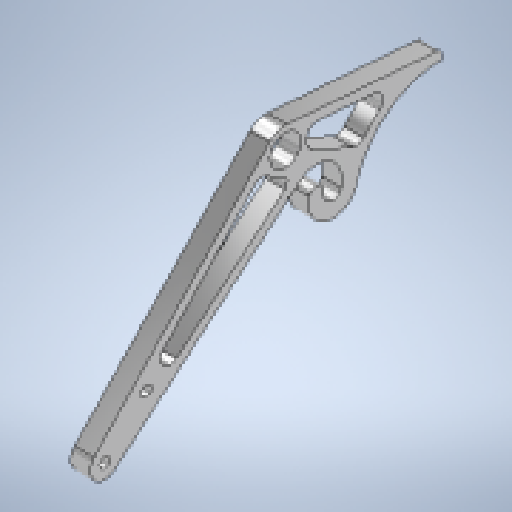
# Autodesk Inventor part: Arm
Saved by Autodesk Inventor 2023.2 (Build 272271000, 271)
## iProperties
Created: 2023-08-22
Part Number: Arm
Material: Aluminum 6061
Document SubType Name: Modeling
Designer: Nathan Cai
Mass: 24.1301 g
Surface Area: 65.2263 cm^2
Volume: 8.93708 cm^3
Density: 2.7 g/cm^3
Appearance: Aluminum - Flat
Author: Nathan Cai
Autodesk Inventor part; units mm, degrees
ref_plane "YZ Plane" through (0, 0, 0) normal (1, 0, 0) x (0, 1, 0)
ref_plane "XZ Plane" through (0, 0, 0) normal (0, 1, 0) x (-1, 0, 0)
ref_plane "XY Plane" through (0, 0, 0) normal (0, 0, 1) x (1, 0, 0)
sketch "Sketch1" plane through (0, 0, 0) normal (1, 0, 0) x (0, 1, 0)
  circle A0 centre (28.575, 50.8) radius 7
  circle A1 centre (0, 0) radius 28.575
  line L0 (0, 0) -> (28.575, 50.8) construction
  line L1 (28.575, 0) -> (-28.575, 0)
  arc A2 (13.9234, 2.1588) -> (28.575, 0) centre (28.575, 50.8) ccw construction
  line L2 (28.575, 0) -> (28.575, 43.8) construction
  circle A3 centre (28.575, 50.8) radius 5
  circle A4 centre (30.1625, 1.5875) radius 1.5875
  line L3 (30.1625, 0) -> (28.575, 0)
  line L4 (31.7452, 1.464) -> (35.5538, 50.2552)
  circle A5 centre (-28.575, 87.3125) radius 3 construction
  line L5 (23.4933, 45.9858) -> (-33.7928, 106.4549) construction
  line L6 (33.3896, 55.8813) -> (-26.8868, 112.9946)
  arc A6 (10.9573, 40.6232) -> (8.0927, 30.0027) centre (9.525, 35.313) ccw construction
  arc A7 (11.6084, 43.0369) -> (7.4416, 27.589) centre (9.525, 35.313) ccw
  arc A8 (10.3063, 38.2094) -> (8.7437, 32.4165) centre (9.525, 35.313) ccw
  arc A9 (10.3063, 38.2094) -> (11.6084, 43.0369) centre (10.9573, 40.6232) ccw
  arc A10 (7.4416, 27.589) -> (8.7437, 32.4165) centre (8.0927, 30.0027) ccw construction
  arc A11 (9.525, 35.313) -> (15.1497, 44.1832) centre (10.9573, 40.6232) ccw construction
  arc A12 (8.7437, 32.4165) -> (17.4365, 46.125) centre (10.9573, 40.6232) ccw
  arc A13 (10.3063, 38.2094) -> (12.863, 42.2414) centre (10.9573, 40.6232) ccw
  arc A14 (10.3063, 38.2094) -> (8.7437, 32.4165) centre (9.525, 35.313) ccw
  arc A15 (17.4365, 46.125) -> (12.863, 42.2414) centre (15.1497, 44.1832) ccw construction
  line L7 (17.4365, 46.125) -> (-33.7928, 106.4549)
  line L8 (9.525, 35.313) -> (-28.575, 87.3125) construction
  arc A16 (-26.8868, 112.9946) -> (-33.7928, 106.4549) centre (-30.1625, 109.5375) ccw
  line L9 (-25.4, 109.5375) -> (-34.925, 109.5375) construction
  circle A17 centre (-30.1625, 109.5375) radius 1.7526
  line L10 (28.575, 50.8) -> (-30.1625, 109.5375) construction
  circle A18 centre (-16.6921, 96.0671) radius 1.7526
  circle A19 centre (-16.6921, 96.0671) radius 5.2756
  line L11 (26.9502, 57.6088) -> (-11.7344, 94.2634)
  line L12 (-16.3371, 90.8034) -> (17.5275, 50.9231)
  arc A20 (17.5275, 50.9231) -> (21.6861, 52.0419) centre (19.3426, 52.4644) ccw
  line L13 (29.3849, 12.0246) -> (31.9322, 44.6576)
  arc A21 (29.3849, 12.0246) -> (2.4085, 31.6585) centre (0, 0) ccw
  arc A22 (31.7234, 1.2983) -> (31.6845, 2.0389) centre (0, 0) ccw
  line L14 (17.3128, 26.6145) -> (25.6201, 44.4543)
  circle A23 centre (20.102, 36.3649) radius 1.5875 construction
  line L15 (10.9573, 40.6232) -> (20.102, 36.3649) construction
  point P0 (-20.3953, 106.8437)
  point P1 (8.7437, 32.4165)
  point P2 (7.4416, 27.589)
  point P3 (12.863, 42.2414)
  dimension "d0" = 14
  dimension "d1" = 57.15
  dimension "d3" = 50.8
  dimension "d4" = 10
  dimension "d5" = 3.175
  dimension "d6" = 6
  dimension "d13" = 2.5
  dimension "d15" = 19.05
  dimension "d21" = 3
  dimension "d25" = 57.15
  dimension "d30" = 9.525
  dimension "d33" = 63.5
  dimension "d34" = 22.225
  dimension "d35" = 64.4637
  dimension "d36" = 3.5052
  dimension "d37" = 45
  dimension "d40" = 19.05
  dimension "d45" = 3.175
  dimension "d46" = 3.175
  dimension "d47" = 4.7625
  dimension "d48" = 3.175
  dimension "d50" = 3.175
  dimension "d51" = 3.175
  constraints: 43 point on circle, 32 end point, 24 tangent, 23 centre point, 6 coincident, 4 point on line, 3 midpoint, 3 perpendicular, 1 horizontal, 1 parallel, 17 other
  measures "d1" diameter of A1
  measures "d3" vertical distance of point (0, 0) L0.end
  measures "d4" diameter of A3
  measures "d5" diameter of A4
  measures "d6" diameter of A5
  measures "d13" radius of A9
  measures "d15" horizontal distance of L10.start L8.start
  measures "d21" radius of A8
  measures "d25" horizontal distance of L10.start L8.end
  measures "d30" diameter of A16
  measures "d33" horizontal distance of L10.start L9.end
  measures "d34" distance from line of L9 L8.end
  measures "d35" distance of L8.start L8.end
  measures "d36" diameter of A17
  measures "d37" angle of L2 L10
  measures "d40" distance of L10.end A18.centre
  measures "d45" distance between parallel lines of L6 L11
  measures "d46" distance between parallel lines of L7 L12
  measures "d47" diameter of A20
  measures "d48" distance between parallel lines of L4 L13
  measures "d50" radial gap between concentric circles of A1 A21
  measures "d51" diameter of A23
extrude "Extrusion1" add sketch "Sketch1" along normal blind 6.35 contours A0 | A0 L11 A19 L6 | L4 A4 L3 A1 A7 A21 L13 A0 | A19 L12 A20 A0 L14 A21 A7 A9 A8 A12 L7 A16 L6 | A19 | A4 A22 | A4 A22
fillet "Fillet2" radius 3.175 7 edges at (3.175, 29.3849, 12.0246) (3.175, 17.3128, 26.6145) (3.175, 31.9322, 44.6576) (3.175, 26.9502, 57.6088) (3.175, -11.7344, 94.2634) (3.175, -16.3371, 90.8034) (3.175, 25.6201, 44.4543)
body "Solid1"
